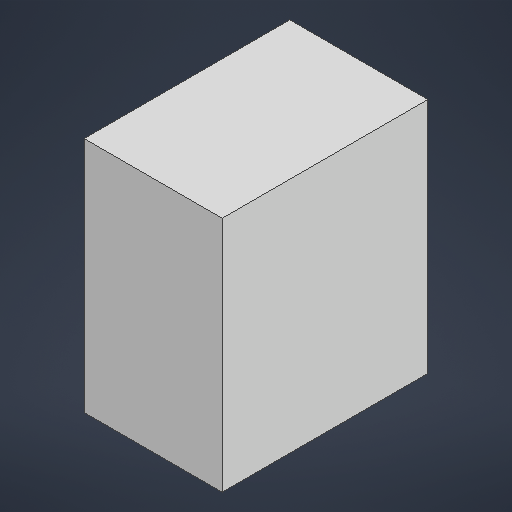
# Autodesk Inventor part: Supporto_magnete
Saved by Autodesk Inventor 2027 (Build 310192060, 192F)
## iProperties
Created: 2026-07-02
Part Number: Supporto_magnete
Material: Generic
Document SubType Name: Modeling
Designer: loren
Density: 1 g/cm^3
Appearance: Default
Author: loren
Autodesk Inventor part; units mm, degrees
ref_plane "YZ Plane" through (0, 0, 0) normal (1, 0, 0) x (0, 1, 0)
ref_plane "XZ Plane" through (0, 0, 0) normal (0, 1, 0) x (-1, 0, 0)
ref_plane "XY Plane" through (0, 0, 0) normal (0, 0, 1) x (1, 0, 0)
sketch "Sketch1" plane through (0, 0, 0) normal (0, 1, 0) x (-1, 0, 0)
  line L0 (-5.82, 8.67) -> (5.82, 8.67)
  line L1 (5.82, 8.67) -> (5.82, -8.67)
  line L2 (5.82, -8.67) -> (-5.82, -8.67)
  line L3 (-5.82, -8.67) -> (-5.82, 8.67)
  line L4 (-5.82, 8.67) -> (5.82, -8.67) construction
  line L5 (5.82, 8.67) -> (-5.82, -8.67) construction
  point P0 (0, 0)
  dimension "d0" = 11.64
  dimension "d1" = 17.34
  constraints: 12 end point, 2 midpoint, 2 parallel, 1 horizontal, 1 perpendicular
  measures "d0" distance of L1.end L2.end
  measures "d1" distance of L0.end L1.end
extrude "Extrusion1" add sketch "Sketch1" along normal blind 20
body "Solid1"
